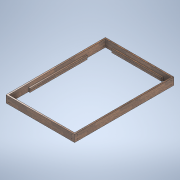
# Autodesk Inventor part: tub floor 1
Saved by Autodesk Inventor 2020 (Build 240168000, 168)
## iProperties
Created: 2020-06-26
Part Number: tub floor 1
Material: Generic
Document SubType Name: Modeling
Designer: Abbas
Density: 1 g/cm^3
Appearance: Default
Author: Abbas
Autodesk Inventor part; units mm, degrees
ref_plane "YZ Plane" through (0, 0, 0) normal (1, 0, 0) x (0, 1, 0)
ref_plane "XZ Plane" through (0, 0, 0) normal (0, 1, 0) x (-1, 0, 0)
ref_plane "XY Plane" through (0, 0, 0) normal (0, 0, 1) x (1, 0, 0)
sketch "Sketch1" plane through (0, 0, 0) normal (0, 1, 0) x (-1, 0, 0)
  line L0 (478.912, 694) -> (-478.912, 694)
  line L1 (-478.912, 694) -> (-478.912, -694)
  line L2 (-478.912, -694) -> (478.912, -694)
  line L3 (478.912, -694) -> (478.912, 694)
  line L4 (478.912, 694) -> (-478.912, -694) construction
  line L5 (-478.912, 694) -> (478.912, -694) construction
  line L6 (458.912, 674) -> (-458.912, 674)
  line L7 (-458.912, 674) -> (-458.912, -674)
  line L8 (-458.912, -674) -> (458.912, -674)
  line L9 (458.912, -674) -> (458.912, 674)
  line L10 (458.912, 674) -> (-458.912, -674) construction
  line L11 (-458.912, 674) -> (458.912, -674) construction
  line L12 (438.912, 400) -> (458.912, 400)
  line L13 (458.912, 400) -> (458.912, -400)
  line L14 (458.912, -400) -> (438.912, -400)
  line L15 (438.912, -400) -> (438.912, 400)
  line L16 (438.912, 400) -> (458.912, -400) construction
  line L17 (458.912, 400) -> (438.912, -400) construction
  line L18 (-458.912, 400) -> (-438.912, 400)
  line L19 (-438.912, 400) -> (-438.912, -400)
  line L20 (-438.912, -400) -> (-458.912, -400)
  line L21 (-458.912, -400) -> (-458.912, 400)
  line L22 (-458.912, 400) -> (-438.912, -400) construction
  line L23 (-438.912, 400) -> (-458.912, -400) construction
  line L24 (-350, 674) -> (350, 674)
  line L25 (350, 674) -> (350, 654)
  line L26 (350, 654) -> (-350, 654)
  line L27 (-350, 654) -> (-350, 674)
  line L28 (-350, 674) -> (350, 654) construction
  line L29 (350, 674) -> (-350, 654) construction
  line L30 (350, -654) -> (-350, -654)
  line L31 (-350, -654) -> (-350, -674)
  line L32 (-350, -674) -> (350, -674)
  line L33 (350, -674) -> (350, -654)
  line L34 (350, -654) -> (-350, -674) construction
  line L35 (-350, -654) -> (350, -674) construction
  point P0 (0, 0)
  point P1 (448.912, 0)
  point P2 (458.912, 0)
  point P3 (-448.912, 0)
  point P4 (-458.912, 0)
  point P5 (0, 664)
  point P6 (0, -664)
  point P7 (0, 674)
  point P8 (0, -674)
  dimension "d0" = 957.824
  dimension "d1" = 1388
  dimension "d2" = 917.824
  dimension "d3" = 1348
  dimension "d4" = 20
  dimension "d5" = 800
  dimension "d6" = 20
  dimension "d7" = 800
  dimension "d8" = 700
  dimension "d9" = 20
  dimension "d10" = 700
  dimension "d11" = 20
  constraints: 72 end point, 20 midpoint, 12 parallel, 6 horizontal, 6 perpendicular, 4 collinear
  measures "d0" distance of L2.end L1.end
  measures "d1" distance of L1.end L0.end
  measures "d2" distance of L8.end L7.end
  measures "d3" distance of L7.end L6.end
  measures "d4" distance of L13.end L14.end
  measures "d5" distance of L12.end L13.end
  measures "d6" distance of L19.end L20.end
  measures "d7" distance of L18.end L19.end
  measures "d8" distance of L25.end L26.end
  measures "d9" distance of L24.end L25.end
  measures "d10" distance of L32.end L31.end
  measures "d11" distance of L31.end L30.end
extrude "Extrusion6" add sketch "Sketch1" along normal blind 50 contours L25 L26 L27 L6 | L9 L14 L15 L12 | L18 L19 L20 L7 | L8 L31 L30 L33
extrude "Extrusion7" add sketch "Sketch1" along normal blind 100
sketch "Sketch2" plane through (478.912, 0, 694) normal (1, 0, 0) x (0, 0, -1)
  line L0 (0, 0) -> (0, 100) projected
  line L1 (0, 100) -> (1388, 100) projected
  point P0 (694, 0)
  point P1 (40, 75)
  dimension "d40" = 40
  dimension "d41" = 25
  measures "d40" distance from line of L0 point (40, 75)
  measures "d41" distance from line of L1 point (40, 75)
hole "Hole1" at (478.912, 75, 654) direction (-1, 0, 0) diameter 8 end through all
sketch "Sketch3" plane through (478.912, 0, 694) normal (1, 0, 0) x (0, 0, -1)
  line L0 (0, 0) -> (0, 100) projected
  line L1 (0, 0) -> (1388, 0) projected
  point P0 (694, 0)
  point P1 (40, 25)
  dimension "d42" = 40
  dimension "d43" = 25
  measures "d42" distance from line of L0 point (40, 25)
  measures "d43" distance from line of L1 point (40, 25)
hole "Hole2" at (478.912, 25, 654) direction (-1, 0, 0) diameter 8 end through all
sketch "Sketch4" plane through (478.912, 0, 694) normal (1, 0, 0) x (0, 0, -1)
  line L0 (1388, 0) -> (1388, 100) projected
  line L1 (0, 100) -> (1388, 100) projected
  point P0 (694, 0)
  point P1 (1348, 75)
  dimension "d58" = 40
  dimension "d59" = 25
  measures "d58" distance from line of L0 point (1348, 75)
  measures "d59" distance from line of L1 point (1348, 75)
hole "Hole3" at (478.912, 75, -654) direction (-1, 0, 0) diameter 8 end through all
sketch "Sketch5" plane through (478.912, 0, 694) normal (1, 0, 0) x (0, 0, -1)
  line L0 (1388, 0) -> (1388, 100) projected
  line L1 (0, 0) -> (1388, 0) projected
  point P0 (694, 0)
  point P1 (1348, 25)
  dimension "d60" = 40
  dimension "d61" = 25
  measures "d60" distance from line of L0 point (1348, 25)
  measures "d61" distance from line of L1 point (1348, 25)
hole "Hole4" at (478.912, 25, -654) direction (-1, 0, 0) diameter 8 end through all
sketch "Sketch6" plane through (-478.912, 0, 694) normal (0, 0, 1) x (1, 0, 0)
  line L0 (0, 100) -> (957.824, 100) projected
  line L1 (957.824, 0) -> (957.824, 100) projected
  line L2 (0, 0) -> (957.824, 0) projected
  point P0 (478.912, 0)
  point P1 (917.824, 75)
  point P2 (917.824, 25)
  dimension "d69" = 25
  dimension "d70" = 40
  dimension "d71" = 40
  dimension "d72" = 25
  measures "d69" distance from line of L0 point (917.824, 75)
  measures "d70" distance from line of L1 point (917.824, 75)
  measures "d71" distance from line of L1 point (917.824, 25)
  measures "d72" distance from line of L2 point (917.824, 25)
hole "Hole5" at (438.912, 75, 694) at (438.912, 25, 694) direction (0, 0, -1) diameter 8 end through all
sketch "Sketch7" plane through (-478.912, 0, 694) normal (0, 0, 1) x (1, 0, 0)
  line L0 (0, 0) -> (0, 100) projected
  line L1 (0, 100) -> (957.824, 100) projected
  point P0 (478.912, 0)
  point P1 (40, 75)
  dimension "d87" = 40
  dimension "d88" = 25
  measures "d87" distance from line of L0 point (40, 75)
  measures "d88" distance from line of L1 point (40, 75)
hole "Hole6" at (-438.912, 75, 694) direction (0, 0, -1) diameter 8 end through all
sketch "Sketch8" plane through (-478.912, 0, 694) normal (0, 0, 1) x (1, 0, 0)
  line L0 (0, 0) -> (0, 100) projected
  line L1 (0, 0) -> (957.824, 0) projected
  point P0 (478.912, 0)
  point P1 (40, 25)
  dimension "d89" = 40
  dimension "d90" = 25
  measures "d89" distance from line of L0 point (40, 25)
  measures "d90" distance from line of L1 point (40, 25)
hole "Hole7" at (-438.912, 25, 694) direction (0, 0, -1) diameter 8 end through all
body "Solid2"
